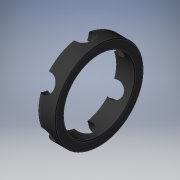
# Autodesk Inventor part: 040102DR-18-H8_cage
Saved by Autodesk Inventor 2024 (Build 280153000, 153)
## iProperties
Created: 2023-06-20
Part Number: 040102DR-18-H8_cage
Material: Generic
Catalog Web Link: www.cadenas.de
Description: DR-H cage-D-Series bearings
Vendor: TOKBEARING
Document SubType Name: Modeling
Designer: psAdmin
Manufacturer: TOKBEARING
Mass: 8700 g
Surface Area: 3.72891 cm^2
Volume: 0.161694 cm^3
Density: 1 g/cm^3
Appearance: PSOLRGB-175-175-175
Category: PARTsolutions
Company: TOKBEARING
PSOL_IDENT_0: {$CADENAS_DATA/23d-libs/tok_bearing/d_series_bearings/dr_h/dr_h_cage.prj},183 {VTYP=3D},{NB=040102DR
PSOL_IDENT_1: -18-H8_cage},{LINA=040102DR-18-H8_cage},{NN=DR-H cage},{DATE=16.12.2020 00:38:04},{GEOMDATE=03.12.20
PSOL_IDENT_2: 12 14:40:00},{VERSION=},{LINEID=1710},{WBVAR=},{WBNUMERIC=}  {NB=040102DR-18-H8_cage},{LINA=040102DR
PSOL_IDENT_3: -18-H8_cage},{KT=DUMMY},{IDNR=},{CODE=040102},{PN=DR-18-H8},{D=18},{SD=8.0},{W=5},{W1=-},{W1X=0.000}
PSOL_IDENT_4: ,{W2=-},{W2X=0.000},{LOAD=49 (5)},{TYPE=11},{QTY=3.000},{GW=8.7},{BD=3.2},{OP=42.704},{N=6},{R=6.8},
PSOL_IDENT_5: {GP=1.4}
NB: 040102DR-18-H8_cage
NN: DR-H cage
NT: D-Series bearings
NBSYN: $CODE.$PN._cage
LINA: 040102DR-18-H8_cage
CATALOG: TOK, Inc
CODE: 040102
PN: DR-18-H8
D: 18
SD: 8
W: 5
W1: -
W2: -
LOAD: 49 (5)
TYPE: 11
QTY: 3.000
GW: 8.7
SUPPLIER: TOKBEARING
ARTICLENO: 040102DR-18-H8_cage
BOMINFO: 040102DR-18-H8_cage
CREATOR: CADENAS GmbH
Title: 040102DR-18-H8_cage
Author: Cadenas PARTsolutions
Comments: D-Series bearings
Autodesk Inventor part; units mm, degrees
sketch "Sketch_1" plane through (0, 0, 0) normal (0, 0, 1) x (1, 0, 0)
  line L0 (5, 0) -> (1.75, 0)
  arc A0 (1.75, 6.1667) -> (1.9167, 6) centre (1.9167, 6.1667) ccw
  line L1 (1.9167, 6) -> (4.8333, 6)
  arc A1 (4.8333, 6) -> (5, 6.1667) centre (4.8333, 6.1667) ccw
  line L2 (5, 6.1667) -> (5, 7.4333)
  arc A2 (5, 7.4333) -> (4.8333, 7.6) centre (4.8333, 7.4333) ccw
  line L3 (4.8333, 7.6) -> (2.4643, 7.6)
  arc A3 (2.4643, 7.6) -> (1.75, 6.8857) centre (2.4643, 6.8857) ccw
  line L4 (1.75, 6.8857) -> (1.75, 6.1667)
  constraints: 10 end point, 8 point on circle, 4 centre point
revolve "Revolution1" add sketch "Sketch_1" angle 360 about axis through (5, 0, 0) along (1, 0, 0)
sketch "Sketch_2" plane through (2.5, 0, 0) normal (1, 0, 0) x (0, 0, -1)
  line L0 (0, 8.4) -> (0, 5.2)
  arc A0 (0, 8.4) -> (0, 5.2) centre (0, 6.8) ccw
  line L1 (0, 8.4) -> (0, 5.2)
  constraints: 4 end point, 2 point on circle, 1 centre point
revolve "Revolution2" cut sketch "Sketch_2" angle 360 about axis through (2.5, 8.4, 0) along (0, 1, 0)
pattern_linear "Rectangular Pattern1" count 3 spacing 6.8 along (0, -0.5, 0.866) count 3 spacing 6.8 along (0, -0.5, -0.866) of "Revolution2"
ref_plane "Cage_OR_XY" through (0, 0, 0) normal (1, 0, 0) x (0, 0, -1)
ref_plane "Cage_OR_YZ" through (0, 0, 0) normal (0, 0, -1) x (0, 1, 0)
ref_plane "Cage_OR_ZX" through (0, 0, 0) normal (0, 1, 0) x (1, 0, 0)
body "Solid1"
